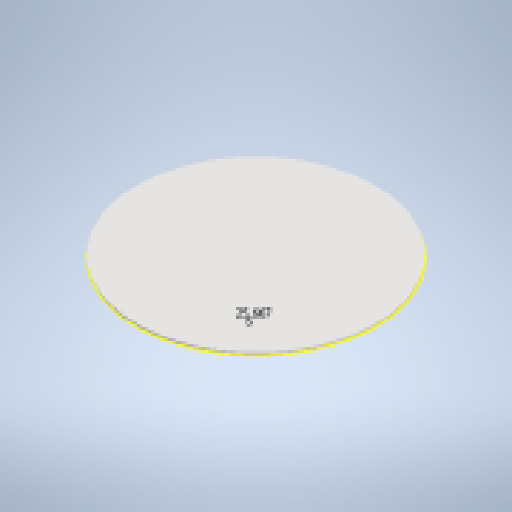
# Autodesk Inventor part: Osn. platform
Saved by Autodesk Inventor 2023.1 (Build 271208000, 208)
## iProperties
Created: 2023-03-13
Part Number: Osn. platform
Material: Типовые
Document SubType Name: Modeling
Designer: User
Density: 1 g/cm^3
Appearance: По умолчанию
Author: User
Autodesk Inventor part; units mm, degrees
ref_plane "YZ Plane" through (0, 0, 0) normal (1, 0, 0) x (0, 1, 0)
ref_plane "XZ Plane" through (0, 0, 0) normal (0, 1, 0) x (-1, 0, 0)
ref_plane "XY Plane" through (0, 0, 0) normal (0, 0, 1) x (1, 0, 0)
sketch "Основ. платформа" plane through (0, 0, 0) normal (0, 1, 0) x (-1, 0, 0)
  circle A0 centre (0, 0) radius 240
  dimension "d117" = 480
  constraints: 1 centre point, 1 coincident
  measures "d117" diameter of A0
extrude "Осн. платформа" add sketch "Основ. платформа" along normal blind 5
sketch "Эскиз13" plane through (0, 0, 0) normal (0, -1, 0) x (1, 0, 0)
  line L0 (0, 0) -> (172.9676, 166.3798) construction
  circle A0 centre (0, 0) radius 240 projected
  line L1 (0, 240) -> (240, 0) construction
  line L2 (104.4061, 0) -> (104.4061, 216.1003) construction
  line L3 (0, 100.4296) -> (217.9768, 100.4296) construction
  line L4 (107.4061, 87.5961) -> (101.4061, 87.5961) construction
  line L5 (101.4061, 87.5961) -> (101.4061, 113.2631) construction
  line L6 (101.4061, 113.2631) -> (107.4061, 113.2631) construction
  line L7 (107.4061, 113.2631) -> (107.4061, 87.5961) construction
  point P0 (104.4061, 100.4296)
  dimension "d120" = 6
  dimension "d121" = 25.667
  constraints: 16 end point, 5 point on circle, 2 horizontal, 2 parallel, 1 perpendicular, 1 vertical
  measures "d120" distance of L5.end L6.end
  measures "d121" distance of L4.end L5.end
sketch "Эскиз14" plane through (0, 5, 0) normal (0, 1, 0) x (1, 0, 0)
  line L0 (137.6204, -61.9298) -> (150.9061, -61.9298) projected
  line L1 (150.9061, -61.9298) -> (150.9061, -55.9298) projected
  line L2 (137.6204, -55.9298) -> (150.9061, -55.9298) projected
  line L3 (137.6204, -61.9298) -> (137.6204, -55.9298) projected
  line L4 (111.049, -61.9298) -> (124.3347, -61.9298) projected
  line L5 (124.3347, -61.9298) -> (124.3347, -55.9298) projected
  line L6 (111.049, -55.9298) -> (124.3347, -55.9298) projected
  line L7 (111.049, -61.9298) -> (111.049, -55.9298) projected
  line L8 (84.4776, -61.9298) -> (97.7633, -61.9298) projected
  line L9 (97.7633, -61.9298) -> (97.7633, -55.9298) projected
  line L10 (84.4776, -55.9298) -> (97.7633, -55.9298) projected
  line L11 (84.4776, -61.9298) -> (84.4776, -55.9298) projected
  line L12 (57.9061, -144.9298) -> (71.1919, -144.9298) projected
  line L13 (71.1919, -144.9298) -> (71.1919, -138.9298) projected
  line L14 (57.9061, -138.9298) -> (71.1919, -138.9298) projected
  line L15 (57.9061, -144.9298) -> (57.9061, -138.9298) projected
  line L16 (84.4776, -144.9298) -> (97.7633, -144.9298) projected
  line L17 (97.7633, -144.9298) -> (97.7633, -138.9298) projected
  line L18 (84.4776, -138.9298) -> (97.7633, -138.9298) projected
  line L19 (84.4776, -144.9298) -> (84.4776, -138.9298) projected
  line L20 (111.049, -144.9298) -> (124.3347, -144.9298) projected
  line L21 (124.3347, -144.9298) -> (124.3347, -138.9298) projected
  line L22 (111.049, -138.9298) -> (124.3347, -138.9298) projected
  line L23 (111.049, -144.9298) -> (111.049, -138.9298) projected
  line L24 (137.6204, -144.9298) -> (150.9061, -144.9298) projected
  line L25 (150.9061, -144.9298) -> (150.9061, -138.9298) projected
  line L26 (137.6204, -138.9298) -> (150.9061, -138.9298) projected
  line L27 (137.6204, -144.9298) -> (137.6204, -138.9298) projected
  line L28 (101.4061, -87.5965) -> (101.4061, -113.2631) projected
  line L29 (101.4061, -113.2631) -> (107.4061, -113.2631) projected
  line L30 (107.4061, -113.2631) -> (107.4061, -87.5965) projected
  line L31 (107.4061, -87.5965) -> (101.4061, -87.5965) projected
  line L32 (57.9061, -61.9298) -> (71.1919, -61.9298) projected
  line L33 (71.1919, -61.9298) -> (71.1919, -55.9298) projected
  line L34 (57.9061, -55.9298) -> (71.1919, -55.9298) projected
  line L35 (57.9061, -61.9298) -> (57.9061, -55.9298) projected
  line L36 (-295.6598, 0) -> (443.256, 0) construction
  line L37 (137.6204, 61.9298) -> (150.9061, 61.9298)
  line L38 (150.9061, 61.9298) -> (150.9061, 55.9298)
  line L39 (137.6204, 55.9298) -> (150.9061, 55.9298)
  line L40 (137.6204, 61.9298) -> (137.6204, 55.9298)
  line L41 (111.049, 61.9298) -> (124.3347, 61.9298)
  line L42 (124.3347, 61.9298) -> (124.3347, 55.9298)
  line L43 (111.049, 55.9298) -> (124.3347, 55.9298)
  line L44 (111.049, 61.9298) -> (111.049, 55.9298)
  line L45 (84.4776, 61.9298) -> (97.7633, 61.9298)
  line L46 (97.7633, 61.9298) -> (97.7633, 55.9298)
  line L47 (84.4776, 55.9298) -> (97.7633, 55.9298)
  line L48 (84.4776, 61.9298) -> (84.4776, 55.9298)
  line L49 (57.9061, 144.9298) -> (71.1919, 144.9298)
  line L50 (71.1919, 144.9298) -> (71.1919, 138.9298)
  line L51 (57.9061, 138.9298) -> (71.1919, 138.9298)
  line L52 (57.9061, 144.9298) -> (57.9061, 138.9298)
  line L53 (84.4776, 144.9298) -> (97.7633, 144.9298)
  line L54 (97.7633, 144.9298) -> (97.7633, 138.9298)
  line L55 (84.4776, 138.9298) -> (97.7633, 138.9298)
  line L56 (84.4776, 144.9298) -> (84.4776, 138.9298)
  line L57 (111.049, 144.9298) -> (124.3347, 144.9298)
  line L58 (124.3347, 144.9298) -> (124.3347, 138.9298)
  line L59 (111.049, 138.9298) -> (124.3347, 138.9298)
  line L60 (111.049, 144.9298) -> (111.049, 138.9298)
  line L61 (137.6204, 144.9298) -> (150.9061, 144.9298)
  line L62 (150.9061, 144.9298) -> (150.9061, 138.9298)
  line L63 (137.6204, 138.9298) -> (150.9061, 138.9298)
  line L64 (137.6204, 144.9298) -> (137.6204, 138.9298)
  line L65 (101.4061, 87.5965) -> (101.4061, 113.2631)
  line L66 (101.4061, 113.2631) -> (107.4061, 113.2631)
  line L67 (107.4061, 113.2631) -> (107.4061, 87.5965)
  line L68 (107.4061, 87.5965) -> (101.4061, 87.5965)
  line L69 (57.9061, 61.9298) -> (71.1919, 61.9298)
  line L70 (71.1919, 61.9298) -> (71.1919, 55.9298)
  line L71 (57.9061, 55.9298) -> (71.1919, 55.9298)
  line L72 (57.9061, 61.9298) -> (57.9061, 55.9298)
  point P0 (0, 0)
  constraints: 74 end point, 36 symmetric about line, 1 horizontal
extrude "Выдавливание9" cut sketch "Эскиз14" against normal up to surface (5 mm away)
